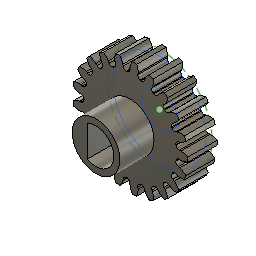
RS6-0845 Gear 21 Teeth HP9000 Laser Fusor v3 (Autodesk Fusion 360 design; units mm, degrees)
description: Spur Gear; Module: 1.024000; Num Teeth: 21; Pressure Angle: 14.500000; Backlash: 0.00 mm
Autodesk Fusion 360 part; units mm, degrees
(part 1 of 3)
sketch "Sketch1" plane through (0, 0, 0) normal (0, 0, 1) x (1, 0, 0) in component "Spur Gear (21 teeth)"
  circle A0 centre (0, 0) radius 9.4724
  circle A1 centre (0, 0) radius 3.625
  dimension "d8" = 7.25
  measures "d8" diameter of A1
extrude "Extrude1" add sketch "Sketch1" along normal blind 4 in component "Spur Gear (21 teeth)"
sketch "Sketch2" plane through (0, 0, 0) normal (0, 0, 1) x (1, 0, 0) in component "Spur Gear (21 teeth)"
  spline S0 degree 5 poles (10.3759, -0.8355) (10.3799, -0.8358) (10.3878, -0.8363) (10.3997, -0.8368) (10.4155, -0.837) (10.4354, -0.8366) (10.4552, -0.8356) (10.4751, -0.8343) (10.495, -0.8328) (10.5149, -0.8312) (10.5348, -0.8295) (10.5547, -0.8276) (10.5746, -0.8256) (10.5946, -0.8232) (10.6145, -0.8207) (10.6345, -0.8178) (10.6544, -0.8148) (10.6744, -0.8116) (10.6943, -0.8083) (10.7143, -0.8048) (10.7343, -0.8012) (10.7542, -0.7975) (10.7742, -0.7936) (10.7942, -0.7895) (10.8142, -0.7853) (10.8341, -0.781) (10.8541, -0.7765) (10.8741, -0.7719) (10.894, -0.7671) (10.914, -0.7622) (10.934, -0.7572) (10.9539, -0.752) (10.9739, -0.7468) (10.9939, -0.7414) (11.0138, -0.7359) (11.0338, -0.7302) (11.0537, -0.7245) (11.0737, -0.7186) (11.0936, -0.7126) (11.1136, -0.7065) (11.1335, -0.7003) (11.1534, -0.694) (11.1733, -0.6875) (11.1933, -0.681) (11.2132, -0.6743) (11.2331, -0.6675) (11.253, -0.6607) (11.2729, -0.6537) (11.2928, -0.6466) (11.3126, -0.6394) (11.3325, -0.6321) (11.3524, -0.6247) (11.3722, -0.6172) (11.3921, -0.6096) (11.4119, -0.6019) (11.4318, -0.5941) (11.4516, -0.5862) (11.4714, -0.5782) (11.4912, -0.5701) (11.511, -0.5619) (11.5308, -0.5536) (11.5506, -0.5452) (11.5704, -0.5367) (11.5901, -0.5281) (11.6099, -0.5194) (11.6296, -0.5106) (11.6494, -0.5018) (11.6691, -0.4928) (11.6888, -0.4838) (11.7085, -0.4746) (11.7282, -0.4654) (11.7439, -0.4579) (11.7557, -0.4523) (11.7636, -0.4485) (11.7675, -0.4466) knots 0 0 0 0 0 0 0.01428571 0.02857143 0.04285714 0.05714286 0.07142857 0.08571429 0.1 0.11428571 0.12857143 0.14285714 0.15714286 0.17142857 0.18571429 0.2 0.21428571 0.22857143 0.24285714 0.25714286 0.27142857 0.28571429 0.3 0.31428571 0.32857143 0.34285714 0.35714286 0.37142857 0.38571429 0.4 0.41428571 0.42857143 0.44285714 0.45714286 0.47142857 0.48571429 0.5 0.51428571 0.52857143 0.54285714 0.55714286 0.57142857 0.58571429 0.6 0.61428571 0.62857143 0.64285714 0.65714286 0.67142857 0.68571429 0.7 0.71428571 0.72857143 0.74285714 0.75714286 0.77142857 0.78571429 0.8 0.81428571 0.82857143 0.84285714 0.85714286 0.87142857 0.88571429 0.9 0.91428571 0.92857143 0.94285714 0.95714286 0.97142857 0.98571429 1 1 1 1 1 1
  spline S1 degree 5 poles (10.3759, 0.8355) (10.3799, 0.8358) (10.3878, 0.8363) (10.3997, 0.8368) (10.4155, 0.837) (10.4354, 0.8366) (10.4552, 0.8356) (10.4751, 0.8343) (10.495, 0.8328) (10.5149, 0.8312) (10.5348, 0.8295) (10.5547, 0.8276) (10.5746, 0.8256) (10.5946, 0.8232) (10.6145, 0.8207) (10.6345, 0.8178) (10.6544, 0.8148) (10.6744, 0.8116) (10.6943, 0.8083) (10.7143, 0.8048) (10.7343, 0.8012) (10.7542, 0.7975) (10.7742, 0.7936) (10.7942, 0.7895) (10.8142, 0.7853) (10.8341, 0.781) (10.8541, 0.7765) (10.8741, 0.7719) (10.894, 0.7671) (10.914, 0.7622) (10.934, 0.7572) (10.9539, 0.752) (10.9739, 0.7468) (10.9939, 0.7414) (11.0138, 0.7359) (11.0338, 0.7302) (11.0537, 0.7245) (11.0737, 0.7186) (11.0936, 0.7126) (11.1136, 0.7065) (11.1335, 0.7003) (11.1534, 0.694) (11.1733, 0.6875) (11.1933, 0.681) (11.2132, 0.6743) (11.2331, 0.6675) (11.253, 0.6607) (11.2729, 0.6537) (11.2928, 0.6466) (11.3126, 0.6394) (11.3325, 0.6321) (11.3524, 0.6247) (11.3722, 0.6172) (11.3921, 0.6096) (11.4119, 0.6019) (11.4318, 0.5941) (11.4516, 0.5862) (11.4714, 0.5782) (11.4912, 0.5701) (11.511, 0.5619) (11.5308, 0.5536) (11.5506, 0.5452) (11.5704, 0.5367) (11.5901, 0.5281) (11.6099, 0.5194) (11.6296, 0.5106) (11.6494, 0.5018) (11.6691, 0.4928) (11.6888, 0.4838) (11.7085, 0.4746) (11.7282, 0.4654) (11.7439, 0.4579) (11.7557, 0.4523) (11.7636, 0.4485) (11.7675, 0.4466) knots 0 0 0 0 0 0 0.01428571 0.02857143 0.04285714 0.05714286 0.07142857 0.08571429 0.1 0.11428571 0.12857143 0.14285714 0.15714286 0.17142857 0.18571429 0.2 0.21428571 0.22857143 0.24285714 0.25714286 0.27142857 0.28571429 0.3 0.31428571 0.32857143 0.34285714 0.35714286 0.37142857 0.38571429 0.4 0.41428571 0.42857143 0.44285714 0.45714286 0.47142857 0.48571429 0.5 0.51428571 0.52857143 0.54285714 0.55714286 0.57142857 0.58571429 0.6 0.61428571 0.62857143 0.64285714 0.65714286 0.67142857 0.68571429 0.7 0.71428571 0.72857143 0.74285714 0.75714286 0.77142857 0.78571429 0.8 0.81428571 0.82857143 0.84285714 0.85714286 0.87142857 0.88571429 0.9 0.91428571 0.92857143 0.94285714 0.95714286 0.97142857 0.98571429 1 1 1 1 1 1
  arc A0 (11.7675, -0.4466) -> (11.7675, 0.4466) centre (0, 0) ccw
  line L0 (9.4319, -0.7602) -> (10.3759, -0.8355)
  line L1 (9.4319, 0.7602) -> (10.3759, 0.8355)
  line L2 (9.4319, -0.7602) -> (9.4319, 0.7602)
  point P0 (10.4739, -0.8344)
  point P1 (10.5725, -0.8257)
  point P2 (10.6715, -0.8121)
  point P3 (10.7707, -0.7943)
  point P4 (10.8701, -0.7727)
  point P5 (10.9697, -0.7479)
  point P6 (11.0694, -0.7198)
  point P7 (11.1691, -0.6889)
  point P8 (11.269, -0.655)
  point P9 (11.3688, -0.6185)
  point P10 (11.4686, -0.5793)
  point P11 (11.5683, -0.5376)
  point P12 (11.668, -0.4933)
  point P13 (10.4739, 0.8344)
  point P14 (10.5725, 0.8257)
  point P15 (10.6715, 0.8121)
  point P16 (10.7707, 0.7943)
  point P17 (10.8701, 0.7727)
  point P18 (10.9697, 0.7479)
  point P19 (11.0694, 0.7198)
  point P20 (11.1691, 0.6889)
  point P21 (11.269, 0.655)
  point P22 (11.3688, 0.6185)
  point P23 (11.4686, 0.5793)
  point P24 (11.5683, 0.5376)
  point P25 (11.668, 0.4933)
extrude "Extrude2" add sketch "Sketch2" along normal blind 4 in component "Spur Gear (21 teeth)"
fillet "Fillet1" radius 0.62 2 edges at (9.4418, -0.761, 2) (9.4418, 0.761, 2) in component "Spur Gear (21 teeth)"
pattern_circular "C-Pattern1" count 21 over 360 about axis through (0, 0, 0) along (0, 0, 1) of "Extrude2", "Fillet1" in component "Spur Gear (21 teeth)"
sketch "Sketch3" plane through (0, 0, 0) normal (0, 0, 1) x (1, 0, 0) in component "Spur Gear (21 teeth)"
  circle A0 centre (0, 0) radius 10.752 construction
sketch "Sketch1 (2)" plane through (0, 0, 0) normal (0, 0, 1) x (1, 0, 0)
  circle A0 centre (0, 0) radius 3.625
  line L0 (-1.775, 0) -> (-1.775, 3.1607)
  line L1 (-1.775, 0) -> (-1.775, -3.1607)
  point P0 (-3.625, 0)
  dimension "d9" = 1.85
  constraint coincident A0.centre origin
  constraint vertical L0
  constraint coincident A0 L0.end
  constraint vertical L1
  constraint coincident A0 L1.end
  measures "d9" distance of P0 L0.start
extrude "Extrude3" add 1 faces at (2.7368, -6.9731, 4) along direction (0, 0, 1) blind 3 in component "Spur Gear (21 teeth)"
sketch "Sketch2 (2)" plane through (0, 0, 7) normal (0, 0, 1) x (1, 0, 0)
  arc A0 (9.3554, -1.4844) -> (9.3773, -1.3391) centre (0, 0) ccw
  arc A1 (10.0403, -0.8087) -> (9.3773, -1.3391) centre (9.991, -1.4268) ccw
  line L0 (10.0403, -0.8087) -> (10.3759, -0.8355)
  spline S0 degree 5 poles (10.3759, -0.8355) (10.3799, -0.8358) (10.3878, -0.8363) (10.3997, -0.8368) (10.4155, -0.837) (10.4354, -0.8366) (10.4552, -0.8356) (10.4751, -0.8343) (10.495, -0.8328) (10.5149, -0.8312) (10.5348, -0.8295) (10.5547, -0.8276) (10.5746, -0.8256) (10.5946, -0.8232) (10.6145, -0.8207) (10.6345, -0.8178) (10.6544, -0.8148) (10.6744, -0.8116) (10.6943, -0.8083) (10.7143, -0.8048) (10.7343, -0.8012) (10.7542, -0.7975) (10.7742, -0.7936) (10.7942, -0.7895) (10.8142, -0.7853) (10.8341, -0.781) (10.8541, -0.7765) (10.8741, -0.7719) (10.894, -0.7671) (10.914, -0.7622) (10.934, -0.7572) (10.9539, -0.752) (10.9739, -0.7468) (10.9939, -0.7414) (11.0138, -0.7359) (11.0338, -0.7302) (11.0537, -0.7245) (11.0737, -0.7186) (11.0936, -0.7126) (11.1136, -0.7065) (11.1335, -0.7003) (11.1534, -0.694) (11.1733, -0.6875) (11.1933, -0.681) (11.2132, -0.6743) (11.2331, -0.6675) (11.253, -0.6607) (11.2729, -0.6537) (11.2928, -0.6466) (11.3126, -0.6394) (11.3325, -0.6321) (11.3524, -0.6247) (11.3722, -0.6172) (11.3921, -0.6096) (11.4119, -0.6019) (11.4318, -0.5941) (11.4516, -0.5862) (11.4714, -0.5782) (11.4912, -0.5701) (11.511, -0.5619) (11.5308, -0.5536) (11.5506, -0.5452) (11.5704, -0.5367) (11.5901, -0.5281) (11.6099, -0.5194) (11.6296, -0.5106) (11.6494, -0.5018) (11.6691, -0.4928) (11.6888, -0.4838) (11.7085, -0.4746) (11.7282, -0.4654) (11.7439, -0.4579) (11.7557, -0.4523) (11.7636, -0.4485) (11.7675, -0.4466) knots 0 0 0 0 0 0 0.01428571 0.02857143 0.04285714 0.05714286 0.07142857 0.08571429 0.1 0.11428571 0.12857143 0.14285714 0.15714286 0.17142857 0.18571429 0.2 0.21428571 0.22857143 0.24285714 0.25714286 0.27142857 0.28571429 0.3 0.31428571 0.32857143 0.34285714 0.35714286 0.37142857 0.38571429 0.4 0.41428571 0.42857143 0.44285714 0.45714286 0.47142857 0.48571429 0.5 0.51428571 0.52857143 0.54285714 0.55714286 0.57142857 0.58571429 0.6 0.61428571 0.62857143 0.64285714 0.65714286 0.67142857 0.68571429 0.7 0.71428571 0.72857143 0.74285714 0.75714286 0.77142857 0.78571429 0.8 0.81428571 0.82857143 0.84285714 0.85714286 0.87142857 0.88571429 0.9 0.91428571 0.92857143 0.94285714 0.95714286 0.97142857 0.98571429 1 1 1 1 1 1
  arc A2 (11.7675, -0.4466) -> (11.7675, 0.4466) centre (0, 0) ccw
  spline S1 degree 5 poles (11.7675, 0.4466) (11.7636, 0.4485) (11.7557, 0.4523) (11.7439, 0.4579) (11.7282, 0.4654) (11.7085, 0.4746) (11.6888, 0.4838) (11.6691, 0.4928) (11.6494, 0.5018) (11.6296, 0.5106) (11.6099, 0.5194) (11.5901, 0.5281) (11.5704, 0.5367) (11.5506, 0.5452) (11.5308, 0.5536) (11.511, 0.5619) (11.4912, 0.5701) (11.4714, 0.5782) (11.4516, 0.5862) (11.4318, 0.5941) (11.4119, 0.6019) (11.3921, 0.6096) (11.3722, 0.6172) (11.3524, 0.6247) (11.3325, 0.6321) (11.3126, 0.6394) (11.2928, 0.6466) (11.2729, 0.6537) (11.253, 0.6607) (11.2331, 0.6675) (11.2132, 0.6743) (11.1933, 0.681) (11.1733, 0.6875) (11.1534, 0.694) (11.1335, 0.7003) (11.1136, 0.7065) (11.0936, 0.7126) (11.0737, 0.7186) (11.0537, 0.7245) (11.0338, 0.7302) (11.0138, 0.7359) (10.9939, 0.7414) (10.9739, 0.7468) (10.9539, 0.752) (10.934, 0.7572) (10.914, 0.7622) (10.894, 0.7671) (10.8741, 0.7719) (10.8541, 0.7765) (10.8341, 0.781) (10.8142, 0.7853) (10.7942, 0.7895) (10.7742, 0.7936) (10.7542, 0.7975) (10.7343, 0.8012) (10.7143, 0.8048) (10.6943, 0.8083) (10.6744, 0.8116) (10.6544, 0.8148) (10.6345, 0.8178) (10.6145, 0.8207) (10.5946, 0.8232) (10.5746, 0.8256) (10.5547, 0.8276) (10.5348, 0.8295) (10.5149, 0.8312) (10.495, 0.8328) (10.4751, 0.8343) (10.4552, 0.8356) (10.4354, 0.8366) (10.4155, 0.837) (10.3997, 0.8368) (10.3878, 0.8363) (10.3799, 0.8358) (10.3759, 0.8355) knots -1 -1 -1 -1 -1 -1 -0.98571429 -0.97142857 -0.95714286 -0.94285714 -0.92857143 -0.91428571 -0.9 -0.88571429 -0.87142857 -0.85714286 -0.84285714 -0.82857143 -0.81428571 -0.8 -0.78571429 -0.77142857 -0.75714286 -0.74285714 -0.72857143 -0.71428571 -0.7 -0.68571429 -0.67142857 -0.65714286 -0.64285714 -0.62857143 -0.61428571 -0.6 -0.58571429 -0.57142857 -0.55714286 -0.54285714 -0.52857143 -0.51428571 -0.5 -0.48571429 -0.47142857 -0.45714286 -0.44285714 -0.42857143 -0.41428571 -0.4 -0.38571429 -0.37142857 -0.35714286 -0.34285714 -0.32857143 -0.31428571 -0.3 -0.28571429 -0.27142857 -0.25714286 -0.24285714 -0.22857143 -0.21428571 -0.2 -0.18571429 -0.17142857 -0.15714286 -0.14285714 -0.12857143 -0.11428571 -0.1 -0.08571429 -0.07142857 -0.05714286 -0.04285714 -0.02857143 -0.01428571 0 0 0 0 0 0
  line L1 (10.3759, 0.8355) -> (10.0403, 0.8087)
  arc A3 (9.3773, 1.3391) -> (10.0403, 0.8087) centre (9.991, 1.4268) ccw
  arc A4 (9.3773, 1.3391) -> (9.3554, 1.4844) centre (0, 0) ccw
  arc A5 (9.8326, 2.1866) -> (9.3554, 1.4844) centre (9.9677, 1.5815) ccw
  line L2 (9.8326, 2.1866) -> (10.1612, 2.26)
  spline S2 degree 5 poles (10.1612, 2.26) (10.1651, 2.2609) (10.1728, 2.2627) (10.1843, 2.2657) (10.1995, 2.2702) (10.2183, 2.2765) (10.237, 2.2832) (10.2556, 2.2903) (10.2742, 2.2976) (10.2928, 2.305) (10.3113, 2.3125) (10.3298, 2.3202) (10.3482, 2.328) (10.3665, 2.3361) (10.3848, 2.3445) (10.4031, 2.3531) (10.4213, 2.3618) (10.4394, 2.3707) (10.4575, 2.3798) (10.4755, 2.389) (10.4936, 2.3983) (10.5115, 2.4078) (10.5295, 2.4174) (10.5474, 2.4272) (10.5652, 2.4371) (10.583, 2.4471) (10.6008, 2.4573) (10.6185, 2.4676) (10.6362, 2.4781) (10.6538, 2.4886) (10.6714, 2.4993) (10.689, 2.5101) (10.7065, 2.521) (10.724, 2.532) (10.7414, 2.5432) (10.7588, 2.5545) (10.7762, 2.5659) (10.7935, 2.5773) (10.8108, 2.5889) (10.8281, 2.6007) (10.8453, 2.6125) (10.8624, 2.6244) (10.8796, 2.6364) (10.8967, 2.6486) (10.9138, 2.6608) (10.9308, 2.6731) (10.9478, 2.6856) (10.9647, 2.6981) (10.9816, 2.7107) (10.9985, 2.7235) (11.0154, 2.7363) (11.0322, 2.7492) (11.0489, 2.7623) (11.0657, 2.7754) (11.0823, 2.7886) (11.099, 2.8019) (11.1156, 2.8153) (11.1322, 2.8288) (11.1487, 2.8424) (11.1652, 2.856) (11.1817, 2.8698) (11.1981, 2.8837) (11.2145, 2.8976) (11.2309, 2.9116) (11.2472, 2.9257) (11.2635, 2.9399) (11.2797, 2.9542) (11.2959, 2.9686) (11.3121, 2.9831) (11.3282, 2.9976) (11.3443, 3.0122) (11.3572, 3.024) (11.3668, 3.0329) (11.3732, 3.0388) (11.3764, 3.0418) knots 0 0 0 0 0 0 0.01428571 0.02857143 0.04285714 0.05714286 0.07142857 0.08571429 0.1 0.11428571 0.12857143 0.14285714 0.15714286 0.17142857 0.18571429 0.2 0.21428571 0.22857143 0.24285714 0.25714286 0.27142857 0.28571429 0.3 0.31428571 0.32857143 0.34285714 0.35714286 0.37142857 0.38571429 0.4 0.41428571 0.42857143 0.44285714 0.45714286 0.47142857 0.48571429 0.5 0.51428571 0.52857143 0.54285714 0.55714286 0.57142857 0.58571429 0.6 0.61428571 0.62857143 0.64285714 0.65714286 0.67142857 0.68571429 0.7 0.71428571 0.72857143 0.74285714 0.75714286 0.77142857 0.78571429 0.8 0.81428571 0.82857143 0.84285714 0.85714286 0.87142857 0.88571429 0.9 0.91428571 0.92857143 0.94285714 0.95714286 0.97142857 0.98571429 1 1 1 1 1 1
  arc A6 (11.3764, 3.0418) -> (11.1131, 3.8953) centre (0, 0) ccw
  spline S3 degree 5 poles (11.1131, 3.8953) (11.1088, 3.896) (11.1001, 3.8973) (11.0872, 3.8992) (11.07, 3.9017) (11.0484, 3.9047) (11.0269, 3.9076) (11.0054, 3.9105) (10.9839, 3.9132) (10.9625, 3.9159) (10.941, 3.9184) (10.9196, 3.9209) (10.8982, 3.9233) (10.8768, 3.9256) (10.8554, 3.9277) (10.834, 3.9298) (10.8127, 3.9318) (10.7914, 3.9337) (10.7701, 3.9355) (10.7488, 3.9373) (10.7275, 3.9389) (10.7063, 3.9404) (10.6851, 3.9418) (10.6639, 3.9431) (10.6427, 3.9443) (10.6216, 3.9454) (10.6005, 3.9465) (10.5794, 3.9474) (10.5583, 3.9482) (10.5373, 3.9489) (10.5162, 3.9495) (10.4953, 3.95) (10.4743, 3.9504) (10.4534, 3.9507) (10.4324, 3.9508) (10.4116, 3.9509) (10.3907, 3.9509) (10.3699, 3.9507) (10.3491, 3.9504) (10.3283, 3.9501) (10.3076, 3.9496) (10.2869, 3.9489) (10.2662, 3.9482) (10.2456, 3.9474) (10.225, 3.9464) (10.2045, 3.9453) (10.1839, 3.9441) (10.1635, 3.9427) (10.143, 3.9413) (10.1226, 3.9397) (10.1022, 3.938) (10.0819, 3.9361) (10.0616, 3.9341) (10.0414, 3.9319) (10.0212, 3.9296) (10.0011, 3.9272) (9.981, 3.9246) (9.9609, 3.9219) (9.9409, 3.9191) (9.921, 3.9161) (9.9011, 3.9129) (9.8812, 3.9095) (9.8615, 3.9058) (9.8418, 3.9019) (9.8223, 3.8979) (9.8027, 3.8936) (9.7832, 3.8893) (9.7638, 3.8848) (9.7444, 3.8802) (9.7252, 3.8753) (9.7061, 3.8699) (9.691, 3.865) (9.6798, 3.861) (9.6724, 3.8582) (9.6687, 3.8567) knots -1 -1 -1 -1 -1 -1 -0.98571429 -0.97142857 -0.95714286 -0.94285714 -0.92857143 -0.91428571 -0.9 -0.88571429 -0.87142857 -0.85714286 -0.84285714 -0.82857143 -0.81428571 -0.8 -0.78571429 -0.77142857 -0.75714286 -0.74285714 -0.72857143 -0.71428571 -0.7 -0.68571429 -0.67142857 -0.65714286 -0.64285714 -0.62857143 -0.61428571 -0.6 -0.58571429 -0.57142857 -0.55714286 -0.54285714 -0.52857143 -0.51428571 -0.5 -0.48571429 -0.47142857 -0.45714286 -0.44285714 -0.42857143 -0.41428571 -0.4 -0.38571429 -0.37142857 -0.35714286 -0.34285714 -0.32857143 -0.31428571 -0.3 -0.28571429 -0.27142857 -0.25714286 -0.24285714 -0.22857143 -0.21428571 -0.2 -0.18571429 -0.17142857 -0.15714286 -0.14285714 -0.12857143 -0.11428571 -0.1 -0.08571429 -0.07142857 -0.05714286 -0.04285714 -0.02857143 -0.01428571 0 0 0 0 0 0
  line L3 (9.6687, 3.8567) -> (9.3558, 3.7322)
  arc A7 (8.566, 4.0436) -> (9.3558, 3.7322) centre (9.1266, 4.3083) ccw
  arc A8 (8.566, 4.0436) -> (8.5022, 4.176) centre (0, 0) ccw
  arc A9 (8.7512, 4.9877) -> (8.5022, 4.176) centre (9.0587, 4.4493) ccw
  line L4 (8.7512, 4.9877) -> (9.0436, 5.1547)
  spline S4 degree 5 poles (9.0436, 5.1547) (9.0471, 5.1567) (9.0539, 5.1607) (9.064, 5.1669) (9.0772, 5.1757) (9.0934, 5.1872) (9.1092, 5.1992) (9.1249, 5.2115) (9.1405, 5.2239) (9.1561, 5.2364) (9.1715, 5.2491) (9.1869, 5.2619) (9.2022, 5.2748) (9.2174, 5.288) (9.2324, 5.3013) (9.2473, 5.3149) (9.2621, 5.3286) (9.2768, 5.3425) (9.2914, 5.3565) (9.306, 5.3706) (9.3204, 5.3848) (9.3348, 5.3992) (9.3491, 5.4136) (9.3633, 5.4282) (9.3775, 5.443) (9.3915, 5.4578) (9.4055, 5.4728) (9.4194, 5.4878) (9.4332, 5.503) (9.4469, 5.5183) (9.4606, 5.5337) (9.4742, 5.5492) (9.4877, 5.5648) (9.5012, 5.5805) (9.5146, 5.5963) (9.5279, 5.6122) (9.5411, 5.6282) (9.5543, 5.6443) (9.5674, 5.6605) (9.5804, 5.6767) (9.5934, 5.6931) (9.6063, 5.7096) (9.6191, 5.7261) (9.6319, 5.7427) (9.6446, 5.7595) (9.6572, 5.7763) (9.6698, 5.7932) (9.6823, 5.8101) (9.6948, 5.8272) (9.7071, 5.8444) (9.7194, 5.8616) (9.7317, 5.8789) (9.7439, 5.8963) (9.756, 5.9137) (9.768, 5.9313) (9.78, 5.9489) (9.792, 5.9666) (9.8038, 5.9844) (9.8156, 6.0022) (9.8274, 6.0202) (9.8391, 6.0382) (9.8507, 6.0563) (9.8622, 6.0744) (9.8737, 6.0926) (9.8851, 6.1109) (9.8965, 6.1293) (9.9078, 6.1477) (9.9191, 6.1662) (9.9303, 6.1848) (9.9414, 6.2035) (9.9524, 6.2222) (9.9613, 6.2372) (9.9678, 6.2485) (9.9722, 6.2561) (9.9744, 6.2599) knots 0 0 0 0 0 0 0.01428571 0.02857143 0.04285714 0.05714286 0.07142857 0.08571429 0.1 0.11428571 0.12857143 0.14285714 0.15714286 0.17142857 0.18571429 0.2 0.21428571 0.22857143 0.24285714 0.25714286 0.27142857 0.28571429 0.3 0.31428571 0.32857143 0.34285714 0.35714286 0.37142857 0.38571429 0.4 0.41428571 0.42857143 0.44285714 0.45714286 0.47142857 0.48571429 0.5 0.51428571 0.52857143 0.54285714 0.55714286 0.57142857 0.58571429 0.6 0.61428571 0.62857143 0.64285714 0.65714286 0.67142857 0.68571429 0.7 0.71428571 0.72857143 0.74285714 0.75714286 0.77142857 0.78571429 0.8 0.81428571 0.82857143 0.84285714 0.85714286 0.87142857 0.88571429 0.9 0.91428571 0.92857143 0.94285714 0.95714286 0.97142857 0.98571429 1 1 1 1 1 1
  arc A10 (9.9744, 6.2599) -> (9.4712, 6.9979) centre (0, 0) ccw
  spline S5 degree 5 poles (9.4712, 6.9979) (9.4669, 6.9973) (9.4583, 6.9959) (9.4453, 6.994) (9.4281, 6.9912) (9.4067, 6.9878) (9.3852, 6.9842) (9.3638, 6.9806) (9.3425, 6.9769) (9.3212, 6.9731) (9.3, 6.9693) (9.2787, 6.9653) (9.2576, 6.9613) (9.2365, 6.9571) (9.2154, 6.9529) (9.1944, 6.9486) (9.1734, 6.9442) (9.1524, 6.9398) (9.1316, 6.9352) (9.1107, 6.9306) (9.0899, 6.9259) (9.0692, 6.9211) (9.0485, 6.9162) (9.0279, 6.9112) (9.0073, 6.9061) (8.9868, 6.9009) (8.9663, 6.8957) (8.9459, 6.8903) (8.9255, 6.8849) (8.9052, 6.8794) (8.8849, 6.8737) (8.8647, 6.868) (8.8446, 6.8622) (8.8245, 6.8563) (8.8044, 6.8503) (8.7845, 6.8442) (8.7645, 6.838) (8.7447, 6.8318) (8.7249, 6.8254) (8.7052, 6.8189) (8.6855, 6.8123) (8.6659, 6.8056) (8.6464, 6.7988) (8.6269, 6.7919) (8.6075, 6.7849) (8.5882, 6.7778) (8.569, 6.7706) (8.5498, 6.7633) (8.5307, 6.7559) (8.5116, 6.7484) (8.4927, 6.7407) (8.4738, 6.7329) (8.455, 6.725) (8.4363, 6.717) (8.4177, 6.7089) (8.3992, 6.7006) (8.3807, 6.6922) (8.3624, 6.6837) (8.3441, 6.6751) (8.3259, 6.6663) (8.3078, 6.6574) (8.2899, 6.6483) (8.2721, 6.639) (8.2545, 6.6295) (8.237, 6.6198) (8.2195, 6.6101) (8.2022, 6.6002) (8.1849, 6.5902) (8.1678, 6.5801) (8.1508, 6.5697) (8.1342, 6.5589) (8.1212, 6.5498) (8.1117, 6.5426) (8.1055, 6.5377) (8.1024, 6.5353) knots -1 -1 -1 -1 -1 -1 -0.98571429 -0.97142857 -0.95714286 -0.94285714 -0.92857143 -0.91428571 -0.9 -0.88571429 -0.87142857 -0.85714286 -0.84285714 -0.82857143 -0.81428571 -0.8 -0.78571429 -0.77142857 -0.75714286 -0.74285714 -0.72857143 -0.71428571 -0.7 -0.68571429 -0.67142857 -0.65714286 -0.64285714 -0.62857143 -0.61428571 -0.6 -0.58571429 -0.57142857 -0.55714286 -0.54285714 -0.52857143 -0.51428571 -0.5 -0.48571429 -0.47142857 -0.45714286 -0.44285714 -0.42857143 -0.41428571 -0.4 -0.38571429 -0.37142857 -0.35714286 -0.34285714 -0.32857143 -0.31428571 -0.3 -0.28571429 -0.27142857 -0.25714286 -0.24285714 -0.22857143 -0.21428571 -0.2 -0.18571429 -0.17142857 -0.15714286 -0.14285714 -0.12857143 -0.11428571 -0.1 -0.08571429 -0.07142857 -0.05714286 -0.04285714 -0.02857143 -0.01428571 0 0 0 0 0 0
  line L5 (8.1024, 6.5353) -> (7.8401, 6.3241)
  arc A11 (6.9935, 6.3888) -> (7.8401, 6.3241) centre (7.4513, 6.807) ccw
  arc A12 (6.9935, 6.3888) -> (6.8936, 6.4965) centre (0, 0) ccw
  arc A13 (6.8923, 7.3456) -> (6.8936, 6.4965) centre (7.3448, 6.9217) ccw
  line L6 (6.8923, 7.3456) -> (7.1225, 7.5913)
  spline S6 degree 5 poles (7.1225, 7.5913) (7.1252, 7.5942) (7.1305, 7.6001) (7.1384, 7.609) (7.1484, 7.6213) (7.1604, 7.6371) (7.172, 7.6532) (7.1834, 7.6696) (7.1947, 7.686) (7.2058, 7.7026) (7.2169, 7.7192) (7.2278, 7.736) (7.2386, 7.7529) (7.2492, 7.7699) (7.2597, 7.7871) (7.2699, 7.8044) (7.28, 7.8219) (7.2899, 7.8395) (7.2998, 7.8572) (7.3095, 7.875) (7.3191, 7.8928) (7.3287, 7.9108) (7.3381, 7.9288) (7.3474, 7.947) (7.3565, 7.9652) (7.3656, 7.9835) (7.3745, 8.0019) (7.3833, 8.0204) (7.3921, 8.039) (7.4007, 8.0577) (7.4092, 8.0764) (7.4176, 8.0952) (7.426, 8.1141) (7.4342, 8.1331) (7.4423, 8.1521) (7.4504, 8.1713) (7.4583, 8.1904) (7.4661, 8.2097) (7.4739, 8.229) (7.4816, 8.2484) (7.4891, 8.2679) (7.4966, 8.2874) (7.504, 8.307) (7.5113, 8.3267) (7.5185, 8.3464) (7.5256, 8.3662) (7.5326, 8.386) (7.5396, 8.4059) (7.5464, 8.4259) (7.5532, 8.4459) (7.5599, 8.466) (7.5665, 8.4862) (7.573, 8.5064) (7.5794, 8.5266) (7.5858, 8.547) (7.5921, 8.5673) (7.5982, 8.5878) (7.6043, 8.6082) (7.6104, 8.6288) (7.6163, 8.6494) (7.6221, 8.67) (7.6279, 8.6907) (7.6336, 8.7115) (7.6392, 8.7323) (7.6448, 8.7531) (7.6502, 8.774) (7.6556, 8.795) (7.6609, 8.816) (7.6661, 8.837) (7.6712, 8.8582) (7.6763, 8.8793) (7.6802, 8.8963) (7.6832, 8.909) (7.6851, 8.9175) (7.6861, 8.9218) knots 0 0 0 0 0 0 0.01428571 0.02857143 0.04285714 0.05714286 0.07142857 0.08571429 0.1 0.11428571 0.12857143 0.14285714 0.15714286 0.17142857 0.18571429 0.2 0.21428571 0.22857143 0.24285714 0.25714286 0.27142857 0.28571429 0.3 0.31428571 0.32857143 0.34285714 0.35714286 0.37142857 0.38571429 0.4 0.41428571 0.42857143 0.44285714 0.45714286 0.47142857 0.48571429 0.5 0.51428571 0.52857143 0.54285714 0.55714286 0.57142857 0.58571429 0.6 0.61428571 0.62857143 0.64285714 0.65714286 0.67142857 0.68571429 0.7 0.71428571 0.72857143 0.74285714 0.75714286 0.77142857 0.78571429 0.8 0.81428571 0.82857143 0.84285714 0.85714286 0.87142857 0.88571429 0.9 0.91428571 0.92857143 0.94285714 0.95714286 0.97142857 0.98571429 1 1 1 1 1 1
  arc A14 (7.6861, 8.9218) -> (6.9877, 9.4787) centre (0, 0) ccw
  spline S7 degree 5 poles (6.9877, 9.4787) (6.9838, 9.4768) (6.976, 9.473) (6.9642, 9.4673) (6.9485, 9.4596) (6.9291, 9.45) (6.9096, 9.4403) (6.8903, 9.4305) (6.871, 9.4207) (6.8517, 9.4108) (6.8326, 9.4008) (6.8135, 9.3908) (6.7944, 9.3807) (6.7755, 9.3705) (6.7566, 9.3603) (6.7377, 9.35) (6.719, 9.3396) (6.7003, 9.3292) (6.6817, 9.3187) (6.6631, 9.3081) (6.6447, 9.2975) (6.6263, 9.2868) (6.6079, 9.276) (6.5897, 9.2651) (6.5715, 9.2542) (6.5534, 9.2432) (6.5354, 9.2322) (6.5175, 9.221) (6.4996, 9.2098) (6.4818, 9.1986) (6.4641, 9.1872) (6.4465, 9.1758) (6.4289, 9.1643) (6.4115, 9.1528) (6.3941, 9.1411) (6.3768, 9.1294) (6.3596, 9.1176) (6.3425, 9.1058) (6.3255, 9.0939) (6.3085, 9.0818) (6.2917, 9.0698) (6.2749, 9.0576) (6.2583, 9.0453) (6.2417, 9.033) (6.2252, 9.0206) (6.2089, 9.0081) (6.1926, 8.9956) (6.1764, 8.9829) (6.1603, 8.9702) (6.1444, 8.9574) (6.1285, 8.9445) (6.1128, 8.9315) (6.0972, 8.9184) (6.0817, 8.9052) (6.0663, 8.892) (6.051, 8.8786) (6.0359, 8.8652) (6.0208, 8.8516) (6.0059, 8.838) (5.9911, 8.8243) (5.9764, 8.8104) (5.962, 8.7965) (5.9477, 8.7823) (5.9337, 8.768) (5.9198, 8.7536) (5.906, 8.7391) (5.8924, 8.7246) (5.8788, 8.7099) (5.8654, 8.6952) (5.8523, 8.6803) (5.8395, 8.6651) (5.8298, 8.6526) (5.8228, 8.6429) (5.8183, 8.6364) (5.8161, 8.6331) knots -1 -1 -1 -1 -1 -1 -0.98571429 -0.97142857 -0.95714286 -0.94285714 -0.92857143 -0.91428571 -0.9 -0.88571429 -0.87142857 -0.85714286 -0.84285714 -0.82857143 -0.81428571 -0.8 -0.78571429 -0.77142857 -0.75714286 -0.74285714 -0.72857143 -0.71428571 -0.7 -0.68571429 -0.67142857 -0.65714286 -0.64285714 -0.62857143 -0.61428571 -0.6 -0.58571429 -0.57142857 -0.55714286 -0.54285714 -0.52857143 -0.51428571 -0.5 -0.48571429 -0.47142857 -0.45714286 -0.44285714 -0.42857143 -0.41428571 -0.4 -0.38571429 -0.37142857 -0.35714286 -0.34285714 -0.32857143 -0.31428571 -0.3 -0.28571429 -0.27142857 -0.25714286 -0.24285714 -0.22857143 -0.21428571 -0.2 -0.18571429 -0.17142857 -0.15714286 -0.14285714 -0.12857143 -0.11428571 -0.1 -0.08571429 -0.07142857 -0.05714286 -0.04285714 -0.02857143 -0.01428571 0 0 0 0 0 0
  line L7 (5.8161, 8.6331) -> (5.6277, 8.354)
  arc A15 (4.7997, 8.1664) -> (5.6277, 8.354) centre (5.1138, 8.7009) ccw
  arc A16 (4.7997, 8.1664) -> (4.6724, 8.2398) centre (0, 0) ccw
  arc A17 (4.4209, 9.0508) -> (4.6724, 8.2398) centre (4.9783, 8.7791) ccw
  line L8 (4.4209, 9.0508) -> (4.5685, 9.3535)
  spline S8 degree 5 poles (4.5685, 9.3535) (4.5702, 9.357) (4.5736, 9.3642) (4.5784, 9.375) (4.5844, 9.3897) (4.5912, 9.4084) (4.5976, 9.4272) (4.6036, 9.4462) (4.6095, 9.4652) (4.6153, 9.4843) (4.621, 9.5035) (4.6265, 9.5227) (4.6318, 9.542) (4.637, 9.5615) (4.6418, 9.581) (4.6465, 9.6006) (4.651, 9.6202) (4.6553, 9.64) (4.6595, 9.6598) (4.6636, 9.6796) (4.6675, 9.6995) (4.6713, 9.7195) (4.675, 9.7395) (4.6785, 9.7596) (4.6819, 9.7797) (4.6851, 9.7999) (4.6883, 9.8201) (4.6912, 9.8404) (4.6941, 9.8607) (4.6968, 9.8811) (4.6995, 9.9015) (4.702, 9.922) (4.7044, 9.9425) (4.7066, 9.963) (4.7088, 9.9836) (4.7108, 10.0043) (4.7128, 10.0249) (4.7146, 10.0457) (4.7163, 10.0664) (4.7179, 10.0872) (4.7194, 10.108) (4.7208, 10.1289) (4.7221, 10.1498) (4.7233, 10.1707) (4.7243, 10.1917) (4.7253, 10.2127) (4.7262, 10.2337) (4.7269, 10.2548) (4.7276, 10.2759) (4.7282, 10.297) (4.7286, 10.3182) (4.729, 10.3394) (4.7293, 10.3606) (4.7294, 10.3819) (4.7295, 10.4032) (4.7295, 10.4245) (4.7294, 10.4459) (4.7292, 10.4672) (4.7289, 10.4886) (4.7285, 10.5101) (4.728, 10.5315) (4.7274, 10.553) (4.7267, 10.5745) (4.7259, 10.596) (4.7251, 10.6176) (4.7241, 10.6392) (4.7231, 10.6608) (4.722, 10.6824) (4.7207, 10.7041) (4.7194, 10.7257) (4.718, 10.7474) (4.7168, 10.7648) (4.7159, 10.7779) (4.7152, 10.7866) (4.7149, 10.7909) knots 0 0 0 0 0 0 0.01428571 0.02857143 0.04285714 0.05714286 0.07142857 0.08571429 0.1 0.11428571 0.12857143 0.14285714 0.15714286 0.17142857 0.18571429 0.2 0.21428571 0.22857143 0.24285714 0.25714286 0.27142857 0.28571429 0.3 0.31428571 0.32857143 0.34285714 0.35714286 0.37142857 0.38571429 0.4 0.41428571 0.42857143 0.44285714 0.45714286 0.47142857 0.48571429 0.5 0.51428571 0.52857143 0.54285714 0.55714286 0.57142857 0.58571429 0.6 0.61428571 0.62857143 0.64285714 0.65714286 0.67142857 0.68571429 0.7 0.71428571 0.72857143 0.74285714 0.75714286 0.77142857 0.78571429 0.8 0.81428571 0.82857143 0.84285714 0.85714286 0.87142857 0.88571429 0.9 0.91428571 0.92857143 0.94285714 0.95714286 0.97142857 0.98571429 1 1 1 1 1 1
  arc A18 (4.7149, 10.7909) -> (3.8834, 11.1173) centre (0, 0) ccw
  spline S9 degree 5 poles (3.8834, 11.1173) (3.8802, 11.1143) (3.8738, 11.1083) (3.8643, 11.0994) (3.8516, 11.0875) (3.8358, 11.0725) (3.8201, 11.0575) (3.8044, 11.0425) (3.7889, 11.0274) (3.7734, 11.0123) (3.7581, 10.9971) (3.7428, 10.9819) (3.7276, 10.9666) (3.7124, 10.9513) (3.6974, 10.936) (3.6824, 10.9206) (3.6676, 10.9052) (3.6528, 10.8897) (3.6381, 10.8742) (3.6235, 10.8586) (3.609, 10.843) (3.5946, 10.8273) (3.5802, 10.8116) (3.566, 10.7959) (3.5518, 10.7801) (3.5378, 10.7642) (3.5238, 10.7484) (3.51, 10.7324) (3.4962, 10.7165) (3.4825, 10.7005) (3.4689, 10.6844) (3.4555, 10.6683) (3.4421, 10.6521) (3.4288, 10.636) (3.4156, 10.6197) (3.4026, 10.6034) (3.3896, 10.5871) (3.3767, 10.5707) (3.364, 10.5543) (3.3513, 10.5378) (3.3388, 10.5213) (3.3264, 10.5048) (3.3141, 10.4881) (3.3019, 10.4715) (3.2898, 10.4548) (3.2778, 10.438) (3.266, 10.4212) (3.2542, 10.4044) (3.2426, 10.3875) (3.2312, 10.3705) (3.2198, 10.3535) (3.2086, 10.3365) (3.1975, 10.3194) (3.1866, 10.3022) (3.1758, 10.285) (3.1652, 10.2677) (3.1546, 10.2504) (3.1443, 10.233) (3.134, 10.2156) (3.1239, 10.1981) (3.114, 10.1806) (3.1043, 10.163) (3.0949, 10.1453) (3.0856, 10.1275) (3.0766, 10.1096) (3.0677, 10.0917) (3.059, 10.0738) (3.0503, 10.0558) (3.0419, 10.0378) (3.0337, 10.0196) (3.026, 10.0013) (3.0204, 9.9865) (3.0166, 9.9753) (3.0142, 9.9677) (3.0131, 9.9639) knots -1 -1 -1 -1 -1 -1 -0.98571429 -0.97142857 -0.95714286 -0.94285714 -0.92857143 -0.91428571 -0.9 -0.88571429 -0.87142857 -0.85714286 -0.84285714 -0.82857143 -0.81428571 -0.8 -0.78571429 -0.77142857 -0.75714286 -0.74285714 -0.72857143 -0.71428571 -0.7 -0.68571429 -0.67142857 -0.65714286 -0.64285714 -0.62857143 -0.61428571 -0.6 -0.58571429 -0.57142857 -0.55714286 -0.54285714 -0.52857143 -0.51428571 -0.5 -0.48571429 -0.47142857 -0.45714286 -0.44285714 -0.42857143 -0.41428571 -0.4 -0.38571429 -0.37142857 -0.35714286 -0.34285714 -0.32857143 -0.31428571 -0.3 -0.28571429 -0.27142857 -0.25714286 -0.24285714 -0.22857143 -0.21428571 -0.2 -0.18571429 -0.17142857 -0.15714286 -0.14285714 -0.12857143 -0.11428571 -0.1 -0.08571429 -0.07142857 -0.05714286 -0.04285714 -0.02857143 -0.01428571 0 0 0 0 0 0
  line L9 (3.0131, 9.9639) -> (2.9153, 9.6417)
  arc A19 (2.1794, 9.2183) -> (2.9153, 9.6417) centre (2.322, 9.8216) ccw
  arc A20 (2.1794, 9.2183) -> (2.0361, 9.251) centre (0, 0) ccw
  arc A21 (1.5568, 9.9518) -> (2.0361, 9.251) centre (2.1694, 9.8565) ccw
  line L10 (1.5568, 9.9518) -> (1.6085, 10.2845)
  spline S10 degree 5 poles (1.6085, 10.2845) (1.6091, 10.2884) (1.6102, 10.2963) (1.6117, 10.3081) (1.6131, 10.3238) (1.6141, 10.3437) (1.6146, 10.3635) (1.6148, 10.3835) (1.6148, 10.4034) (1.6147, 10.4234) (1.6145, 10.4433) (1.6141, 10.4634) (1.6135, 10.4834) (1.6127, 10.5034) (1.6116, 10.5235) (1.6103, 10.5436) (1.6088, 10.5637) (1.6071, 10.5839) (1.6052, 10.604) (1.6033, 10.6242) (1.6012, 10.6444) (1.5989, 10.6646) (1.5965, 10.6848) (1.594, 10.705) (1.5913, 10.7252) (1.5884, 10.7455) (1.5854, 10.7657) (1.5823, 10.786) (1.5791, 10.8063) (1.5757, 10.8265) (1.5722, 10.8468) (1.5685, 10.8671) (1.5648, 10.8874) (1.5609, 10.9077) (1.5569, 10.928) (1.5527, 10.9483) (1.5485, 10.9687) (1.5441, 10.989) (1.5396, 11.0093) (1.535, 11.0297) (1.5303, 11.05) (1.5255, 11.0704) (1.5206, 11.0907) (1.5155, 11.1111) (1.5104, 11.1314) (1.5051, 11.1518) (1.4997, 11.1721) (1.4943, 11.1925) (1.4887, 11.2129) (1.483, 11.2332) (1.4772, 11.2536) (1.4713, 11.274) (1.4653, 11.2943) (1.4592, 11.3147) (1.453, 11.3351) (1.4467, 11.3554) (1.4403, 11.3758) (1.4338, 11.3961) (1.4272, 11.4165) (1.4205, 11.4369) (1.4137, 11.4572) (1.4068, 11.4776) (1.3998, 11.4979) (1.3928, 11.5183) (1.3856, 11.5386) (1.3783, 11.559) (1.3709, 11.5793) (1.3635, 11.5996) (1.3559, 11.62) (1.3483, 11.6403) (1.3405, 11.6606) (1.3343, 11.6769) (1.3295, 11.6891) (1.3264, 11.6972) (1.3248, 11.7012) knots 0 0 0 0 0 0 0.01428571 0.02857143 0.04285714 0.05714286 0.07142857 0.08571429 0.1 0.11428571 0.12857143 0.14285714 0.15714286 0.17142857 0.18571429 0.2 0.21428571 0.22857143 0.24285714 0.25714286 0.27142857 0.28571429 0.3 0.31428571 0.32857143 0.34285714 0.35714286 0.37142857 0.38571429 0.4 0.41428571 0.42857143 0.44285714 0.45714286 0.47142857 0.48571429 0.5 0.51428571 0.52857143 0.54285714 0.55714286 0.57142857 0.58571429 0.6 0.61428571 0.62857143 0.64285714 0.65714286 0.67142857 0.68571429 0.7 0.71428571 0.72857143 0.74285714 0.75714286 0.77142857 0.78571429 0.8 0.81428571 0.82857143 0.84285714 0.85714286 0.87142857 0.88571429 0.9 0.91428571 0.92857143 0.94285714 0.95714286 0.97142857 0.98571429 1 1 1 1 1 1
  arc A22 (1.3248, 11.7012) -> (0.434, 11.768) centre (0, 0) ccw
  spline S11 degree 5 poles (0.434, 11.768) (0.4318, 11.7642) (0.4275, 11.7567) (0.421, 11.7453) (0.4124, 11.7302) (0.4017, 11.7112) (0.3911, 11.6923) (0.3806, 11.6733) (0.3702, 11.6543) (0.3599, 11.6353) (0.3496, 11.6163) (0.3395, 11.5972) (0.3295, 11.5781) (0.3195, 11.5591) (0.3097, 11.54) (0.2999, 11.5208) (0.2903, 11.5017) (0.2807, 11.4826) (0.2713, 11.4634) (0.2619, 11.4442) (0.2526, 11.425) (0.2435, 11.4058) (0.2344, 11.3866) (0.2254, 11.3673) (0.2166, 11.3481) (0.2078, 11.3288) (0.1991, 11.3095) (0.1906, 11.2902) (0.1821, 11.2709) (0.1738, 11.2516) (0.1655, 11.2322) (0.1574, 11.2128) (0.1494, 11.1935) (0.1415, 11.1741) (0.1337, 11.1547) (0.126, 11.1353) (0.1184, 11.1158) (0.1109, 11.0964) (0.1036, 11.077) (0.0964, 11.0575) (0.0892, 11.038) (0.0823, 11.0185) (0.0754, 10.999) (0.0686, 10.9795) (0.062, 10.96) (0.0555, 10.9404) (0.0492, 10.9209) (0.0429, 10.9013) (0.0368, 10.8818) (0.0308, 10.8622) (0.025, 10.8426) (0.0193, 10.823) (0.0138, 10.8034) (0.0084, 10.7838) (0.0032, 10.7641) (-0.0019, 10.7445) (-0.0069, 10.7248) (-0.0117, 10.7052) (-0.0163, 10.6855) (-0.0208, 10.6659) (-0.0251, 10.6462) (-0.0292, 10.6265) (-0.033, 10.6068) (-0.0366, 10.5871) (-0.0399, 10.5673) (-0.0431, 10.5476) (-0.0462, 10.5279) (-0.0492, 10.5081) (-0.052, 10.4884) (-0.0544, 10.4687) (-0.0564, 10.4489) (-0.0573, 10.4331) (-0.0577, 10.4213) (-0.0577, 10.4133) (-0.0577, 10.4094) knots -1 -1 -1 -1 -1 -1 -0.98571429 -0.97142857 -0.95714286 -0.94285714 -0.92857143 -0.91428571 -0.9 -0.88571429 -0.87142857 -0.85714286 -0.84285714 -0.82857143 -0.81428571 -0.8 -0.78571429 -0.77142857 -0.75714286 -0.74285714 -0.72857143 -0.71428571 -0.7 -0.68571429 -0.67142857 -0.65714286 -0.64285714 -0.62857143 -0.61428571 -0.6 -0.58571429 -0.57142857 -0.55714286 -0.54285714 -0.52857143 -0.51428571 -0.5 -0.48571429 -0.47142857 -0.45714286 -0.44285714 -0.42857143 -0.41428571 -0.4 -0.38571429 -0.37142857 -0.35714286 -0.34285714 -0.32857143 -0.31428571 -0.3 -0.28571429 -0.27142857 -0.25714286 -0.24285714 -0.22857143 -0.21428571 -0.2 -0.18571429 -0.17142857 -0.15714286 -0.14285714 -0.12857143 -0.11428571 -0.1 -0.08571429 -0.07142857 -0.05714286 -0.04285714 -0.02857143 -0.01428571 0 0 0 0 0 0
  line L11 (-0.0577, 10.4094) -> (-0.0561, 10.0726)
  arc A23 (-0.6346, 9.4511) -> (-0.0561, 10.0726) centre (-0.6761, 10.0697) ccw
  arc A24 (-0.6346, 9.4511) -> (-0.7811, 9.4401) centre (0, 0) ccw
  arc A25 (-1.4457, 9.9685) -> (-0.7811, 9.4401) centre (-0.8322, 10.058) ccw
  line L12 (-1.4457, 9.9685) -> (-1.4944, 10.3017)
  spline S12 degree 5 poles (-1.4944, 10.3017) (-1.4949, 10.3056) (-1.4962, 10.3135) (-1.4983, 10.3251) (-1.5016, 10.3406) (-1.5065, 10.3599) (-1.5118, 10.379) (-1.5175, 10.3981) (-1.5234, 10.4172) (-1.5294, 10.4362) (-1.5355, 10.4553) (-1.5417, 10.4743) (-1.5482, 10.4932) (-1.5549, 10.5121) (-1.5619, 10.531) (-1.5691, 10.5498) (-1.5764, 10.5686) (-1.584, 10.5874) (-1.5917, 10.6061) (-1.5995, 10.6248) (-1.6074, 10.6434) (-1.6155, 10.6621) (-1.6238, 10.6807) (-1.6322, 10.6992) (-1.6407, 10.7178) (-1.6494, 10.7363) (-1.6582, 10.7547) (-1.6672, 10.7732) (-1.6763, 10.7916) (-1.6855, 10.81) (-1.6948, 10.8283) (-1.7043, 10.8466) (-1.7139, 10.8649) (-1.7236, 10.8832) (-1.7334, 10.9014) (-1.7433, 10.9196) (-1.7534, 10.9378) (-1.7635, 10.9559) (-1.7738, 10.974) (-1.7842, 10.9921) (-1.7947, 11.0102) (-1.8053, 11.0282) (-1.816, 11.0462) (-1.8268, 11.0641) (-1.8378, 11.0821) (-1.8488, 11.1) (-1.8599, 11.1179) (-1.8712, 11.1357) (-1.8825, 11.1535) (-1.8939, 11.1713) (-1.9055, 11.189) (-1.9171, 11.2068) (-1.9288, 11.2245) (-1.9407, 11.2421) (-1.9526, 11.2598) (-1.9646, 11.2774) (-1.9768, 11.2949) (-1.989, 11.3125) (-2.0013, 11.33) (-2.0137, 11.3475) (-2.0262, 11.3649) (-2.0388, 11.3823) (-2.0514, 11.3997) (-2.0642, 11.4171) (-2.0771, 11.4344) (-2.09, 11.4517) (-2.103, 11.469) (-2.1162, 11.4862) (-2.1294, 11.5034) (-2.1427, 11.5206) (-2.156, 11.5377) (-2.1668, 11.5514) (-2.1749, 11.5616) (-2.1804, 11.5685) (-2.1831, 11.5719) knots 0 0 0 0 0 0 0.01428571 0.02857143 0.04285714 0.05714286 0.07142857 0.08571429 0.1 0.11428571 0.12857143 0.14285714 0.15714286 0.17142857 0.18571429 0.2 0.21428571 0.22857143 0.24285714 0.25714286 0.27142857 0.28571429 0.3 0.31428571 0.32857143 0.34285714 0.35714286 0.37142857 0.38571429 0.4 0.41428571 0.42857143 0.44285714 0.45714286 0.47142857 0.48571429 0.5 0.51428571 0.52857143 0.54285714 0.55714286 0.57142857 0.58571429 0.6 0.61428571 0.62857143 0.64285714 0.65714286 0.67142857 0.68571429 0.7 0.71428571 0.72857143 0.74285714 0.75714286 0.77142857 0.78571429 0.8 0.81428571 0.82857143 0.84285714 0.85714286 0.87142857 0.88571429 0.9 0.91428571 0.92857143 0.94285714 0.95714286 0.97142857 0.98571429 1 1 1 1 1 1
  arc A26 (-2.1831, 11.5719) -> (-3.0539, 11.3731) centre (0, 0) ccw
  spline S13 degree 5 poles (-3.0539, 11.3731) (-3.0549, 11.3689) (-3.0568, 11.3603) (-3.0597, 11.3476) (-3.0635, 11.3306) (-3.0681, 11.3093) (-3.0726, 11.2881) (-3.0771, 11.2669) (-3.0814, 11.2456) (-3.0857, 11.2244) (-3.0898, 11.2032) (-3.0939, 11.182) (-3.0979, 11.1609) (-3.1018, 11.1397) (-3.1055, 11.1185) (-3.1092, 11.0974) (-3.1128, 11.0763) (-3.1163, 11.0552) (-3.1197, 11.0341) (-3.123, 11.013) (-3.1262, 10.9919) (-3.1293, 10.9708) (-3.1323, 10.9498) (-3.1352, 10.9288) (-3.138, 10.9077) (-3.1407, 10.8867) (-3.1432, 10.8658) (-3.1457, 10.8448) (-3.1481, 10.8238) (-3.1504, 10.8029) (-3.1526, 10.782) (-3.1546, 10.7611) (-3.1566, 10.7402) (-3.1584, 10.7194) (-3.1602, 10.6985) (-3.1618, 10.6777) (-3.1633, 10.6569) (-3.1647, 10.6361) (-3.166, 10.6154) (-3.1672, 10.5946) (-3.1682, 10.5739) (-3.1692, 10.5532) (-3.17, 10.5326) (-3.1707, 10.512) (-3.1712, 10.4913) (-3.1717, 10.4708) (-3.172, 10.4502) (-3.1722, 10.4297) (-3.1723, 10.4092) (-3.1722, 10.3887) (-3.172, 10.3683) (-3.1717, 10.3479) (-3.1712, 10.3275) (-3.1705, 10.3072) (-3.1698, 10.2869) (-3.1688, 10.2666) (-3.1678, 10.2464) (-3.1666, 10.2261) (-3.1652, 10.206) (-3.1637, 10.1859) (-3.162, 10.1658) (-3.1601, 10.1458) (-3.1579, 10.1258) (-3.1555, 10.1059) (-3.1529, 10.0861) (-3.1502, 10.0663) (-3.1473, 10.0465) (-3.1443, 10.0268) (-3.1412, 10.0071) (-3.1377, 9.9876) (-3.1337, 9.9681) (-3.13, 9.9527) (-3.1268, 9.9413) (-3.1246, 9.9337) (-3.1234, 9.9299) knots -1 -1 -1 -1 -1 -1 -0.98571429 -0.97142857 -0.95714286 -0.94285714 -0.92857143 -0.91428571 -0.9 -0.88571429 -0.87142857 -0.85714286 -0.84285714 -0.82857143 -0.81428571 -0.8 -0.78571429 -0.77142857 -0.75714286 -0.74285714 -0.72857143 -0.71428571 -0.7 -0.68571429 -0.67142857 -0.65714286 -0.64285714 -0.62857143 -0.61428571 -0.6 -0.58571429 -0.57142857 -0.55714286 -0.54285714 -0.52857143 -0.51428571 -0.5 -0.48571429 -0.47142857 -0.45714286 -0.44285714 -0.42857143 -0.41428571 -0.4 -0.38571429 -0.37142857 -0.35714286 -0.34285714 -0.32857143 -0.31428571 -0.3 -0.28571429 -0.27142857 -0.25714286 -0.24285714 -0.22857143 -0.21428571 -0.2 -0.18571429 -0.17142857 -0.15714286 -0.14285714 -0.12857143 -0.11428571 -0.1 -0.08571429 -0.07142857 -0.05714286 -0.04285714 -0.02857143 -0.01428571 0 0 0 0 0 0
  line L13 (-3.1234, 9.9299) -> (-3.0226, 9.6086)
  arc A27 (-3.3922, 8.8442) -> (-3.0226, 9.6086) centre (-3.6142, 9.4231) ccw
  arc A28 (-3.3922, 8.8442) -> (-3.5289, 8.7905) centre (0, 0) ccw
  arc A29 (-4.3198, 9.0995) -> (-3.5289, 8.7905) centre (-3.7599, 9.3659) ccw
  line L14 (-4.3198, 9.0995) -> (-4.4645, 9.4036)
  spline S14 degree 5 poles (-4.4645, 9.4036) (-4.4662, 9.4071) (-4.4696, 9.4143) (-4.4751, 9.4248) (-4.4829, 9.4386) (-4.4932, 9.4556) (-4.5039, 9.4723) (-4.515, 9.4889) (-4.5262, 9.5053) (-4.5376, 9.5218) (-4.549, 9.5382) (-4.5606, 9.5545) (-4.5724, 9.5707) (-4.5844, 9.5868) (-4.5966, 9.6028) (-4.609, 9.6186) (-4.6215, 9.6344) (-4.6343, 9.6501) (-4.6472, 9.6657) (-4.6601, 9.6813) (-4.6732, 9.6968) (-4.6865, 9.7122) (-4.6998, 9.7275) (-4.7133, 9.7428) (-4.727, 9.758) (-4.7407, 9.7731) (-4.7546, 9.7882) (-4.7686, 9.8031) (-4.7827, 9.8181) (-4.7969, 9.8329) (-4.8112, 9.8477) (-4.8257, 9.8624) (-4.8402, 9.8771) (-4.8549, 9.8917) (-4.8696, 9.9062) (-4.8845, 9.9206) (-4.8994, 9.935) (-4.9145, 9.9494) (-4.9297, 9.9637) (-4.9449, 9.9779) (-4.9603, 9.992) (-4.9757, 10.0061) (-4.9913, 10.0202) (-5.0069, 10.0341) (-5.0226, 10.048) (-5.0384, 10.0619) (-5.0543, 10.0757) (-5.0703, 10.0894) (-5.0864, 10.1031) (-5.1026, 10.1167) (-5.1189, 10.1303) (-5.1352, 10.1438) (-5.1516, 10.1572) (-5.1681, 10.1706) (-5.1847, 10.184) (-5.2014, 10.1972) (-5.2182, 10.2105) (-5.235, 10.2236) (-5.2519, 10.2367) (-5.2689, 10.2498) (-5.286, 10.2628) (-5.3032, 10.2757) (-5.3204, 10.2886) (-5.3377, 10.3014) (-5.3551, 10.3142) (-5.3726, 10.3269) (-5.3901, 10.3395) (-5.4078, 10.3521) (-5.4254, 10.3647) (-5.4432, 10.3772) (-5.4611, 10.3896) (-5.4754, 10.3995) (-5.4862, 10.4069) (-5.4934, 10.4118) (-5.497, 10.4143) knots 0 0 0 0 0 0 0.01428571 0.02857143 0.04285714 0.05714286 0.07142857 0.08571429 0.1 0.11428571 0.12857143 0.14285714 0.15714286 0.17142857 0.18571429 0.2 0.21428571 0.22857143 0.24285714 0.25714286 0.27142857 0.28571429 0.3 0.31428571 0.32857143 0.34285714 0.35714286 0.37142857 0.38571429 0.4 0.41428571 0.42857143 0.44285714 0.45714286 0.47142857 0.48571429 0.5 0.51428571 0.52857143 0.54285714 0.55714286 0.57142857 0.58571429 0.6 0.61428571 0.62857143 0.64285714 0.65714286 0.67142857 0.68571429 0.7 0.71428571 0.72857143 0.74285714 0.75714286 0.77142857 0.78571429 0.8 0.81428571 0.82857143 0.84285714 0.85714286 0.87142857 0.88571429 0.9 0.91428571 0.92857143 0.94285714 0.95714286 0.97142857 0.98571429 1 1 1 1 1 1
  arc A30 (-5.497, 10.4143) -> (-6.2706, 9.9677) centre (0, 0) ccw
  spline S15 degree 5 poles (-6.2706, 9.9677) (-6.2702, 9.9633) (-6.2696, 9.9546) (-6.2685, 9.9416) (-6.2671, 9.9242) (-6.2653, 9.9025) (-6.2634, 9.8809) (-6.2613, 9.8593) (-6.2592, 9.8378) (-6.2571, 9.8162) (-6.2548, 9.7948) (-6.2524, 9.7733) (-6.25, 9.7519) (-6.2474, 9.7305) (-6.2448, 9.7092) (-6.2421, 9.6879) (-6.2393, 9.6667) (-6.2364, 9.6455) (-6.2334, 9.6243) (-6.2304, 9.6032) (-6.2272, 9.5821) (-6.224, 9.5611) (-6.2206, 9.5401) (-6.2172, 9.5191) (-6.2137, 9.4982) (-6.2101, 9.4773) (-6.2063, 9.4565) (-6.2025, 9.4358) (-6.1986, 9.415) (-6.1946, 9.3944) (-6.1906, 9.3737) (-6.1864, 9.3532) (-6.1821, 9.3326) (-6.1777, 9.3122) (-6.1732, 9.2917) (-6.1686, 9.2714) (-6.1639, 9.251) (-6.1592, 9.2308) (-6.1543, 9.2106) (-6.1493, 9.1904) (-6.1442, 9.1703) (-6.139, 9.1503) (-6.1337, 9.1303) (-6.1283, 9.1104) (-6.1227, 9.0905) (-6.1171, 9.0707) (-6.1113, 9.051) (-6.1055, 9.0313) (-6.0995, 9.0117) (-6.0934, 8.9921) (-6.0872, 8.9727) (-6.0809, 8.9533) (-6.0744, 8.9339) (-6.0678, 8.9147) (-6.061, 8.8955) (-6.0542, 8.8764) (-6.0472, 8.8574) (-6.0401, 8.8385) (-6.0329, 8.8196) (-6.0255, 8.8008) (-6.018, 8.7821) (-6.0102, 8.7636) (-6.0023, 8.7451) (-5.9941, 8.7268) (-5.9858, 8.7086) (-5.9773, 8.6905) (-5.9688, 8.6725) (-5.9601, 8.6545) (-5.9513, 8.6367) (-5.9422, 8.619) (-5.9327, 8.6016) (-5.9246, 8.588) (-5.9182, 8.5779) (-5.9137, 8.5714) (-5.9115, 8.5681) knots -1 -1 -1 -1 -1 -1 -0.98571429 -0.97142857 -0.95714286 -0.94285714 -0.92857143 -0.91428571 -0.9 -0.88571429 -0.87142857 -0.85714286 -0.84285714 -0.82857143 -0.81428571 -0.8 -0.78571429 -0.77142857 -0.75714286 -0.74285714 -0.72857143 -0.71428571 -0.7 -0.68571429 -0.67142857 -0.65714286 -0.64285714 -0.62857143 -0.61428571 -0.6 -0.58571429 -0.57142857 -0.55714286 -0.54285714 -0.52857143 -0.51428571 -0.5 -0.48571429 -0.47142857 -0.45714286 -0.44285714 -0.42857143 -0.41428571 -0.4 -0.38571429 -0.37142857 -0.35714286 -0.34285714 -0.32857143 -0.31428571 -0.3 -0.28571429 -0.27142857 -0.25714286 -0.24285714 -0.22857143 -0.21428571 -0.2 -0.18571429 -0.17142857 -0.15714286 -0.14285714 -0.12857143 -0.11428571 -0.1 -0.08571429 -0.07142857 -0.05714286 -0.04285714 -0.02857143 -0.01428571 0 0 0 0 0 0
  line L15 (-5.9115, 8.5681) -> (-5.7205, 8.2908)
  arc A31 (-5.8483, 7.4514) -> (-5.7205, 8.2908) centre (-6.2311, 7.9391) ccw
  arc A32 (-5.8483, 7.4514) -> (-5.9632, 7.3598) centre (0, 0) ccw
  arc A33 (-6.81, 7.422) -> (-5.9632, 7.3598) centre (-6.3535, 7.8415) ccw
  line L16 (-6.81, 7.422) -> (-7.0379, 7.6699)
  spline S16 degree 5 poles (-7.0379, 7.6699) (-7.0405, 7.6728) (-7.046, 7.6786) (-7.0543, 7.687) (-7.0658, 7.698) (-7.0806, 7.7111) (-7.0958, 7.7239) (-7.1113, 7.7365) (-7.1269, 7.7489) (-7.1426, 7.7613) (-7.1583, 7.7736) (-7.1742, 7.7857) (-7.1902, 7.7978) (-7.2064, 7.8096) (-7.2228, 7.8213) (-7.2393, 7.8328) (-7.256, 7.8442) (-7.2728, 7.8554) (-7.2897, 7.8665) (-7.3067, 7.8776) (-7.3238, 7.8885) (-7.341, 7.8993) (-7.3583, 7.9101) (-7.3757, 7.9207) (-7.3932, 7.9312) (-7.4108, 7.9416) (-7.4285, 7.9519) (-7.4463, 7.9621) (-7.4641, 7.9721) (-7.4821, 7.9821) (-7.5002, 7.992) (-7.5183, 8.0019) (-7.5365, 8.0116) (-7.5548, 8.0212) (-7.5732, 8.0307) (-7.5916, 8.0402) (-7.6102, 8.0495) (-7.6288, 8.0588) (-7.6475, 8.068) (-7.6663, 8.077) (-7.6851, 8.086) (-7.704, 8.095) (-7.723, 8.1038) (-7.7421, 8.1125) (-7.7612, 8.1212) (-7.7804, 8.1298) (-7.7997, 8.1383) (-7.819, 8.1467) (-7.8384, 8.155) (-7.8579, 8.1633) (-7.8774, 8.1714) (-7.897, 8.1795) (-7.9167, 8.1875) (-7.9364, 8.1955) (-7.9562, 8.2033) (-7.976, 8.2111) (-7.9959, 8.2188) (-8.0159, 8.2264) (-8.0359, 8.2339) (-8.056, 8.2414) (-8.0762, 8.2487) (-8.0964, 8.256) (-8.1167, 8.2633) (-8.137, 8.2704) (-8.1574, 8.2775) (-8.1778, 8.2845) (-8.1983, 8.2914) (-8.2188, 8.2983) (-8.2395, 8.305) (-8.2601, 8.3117) (-8.2808, 8.3183) (-8.2974, 8.3236) (-8.3099, 8.3275) (-8.3183, 8.3301) (-8.3224, 8.3313) knots 0 0 0 0 0 0 0.01428571 0.02857143 0.04285714 0.05714286 0.07142857 0.08571429 0.1 0.11428571 0.12857143 0.14285714 0.15714286 0.17142857 0.18571429 0.2 0.21428571 0.22857143 0.24285714 0.25714286 0.27142857 0.28571429 0.3 0.31428571 0.32857143 0.34285714 0.35714286 0.37142857 0.38571429 0.4 0.41428571 0.42857143 0.44285714 0.45714286 0.47142857 0.48571429 0.5 0.51428571 0.52857143 0.54285714 0.55714286 0.57142857 0.58571429 0.6 0.61428571 0.62857143 0.64285714 0.65714286 0.67142857 0.68571429 0.7 0.71428571 0.72857143 0.74285714 0.75714286 0.77142857 0.78571429 0.8 0.81428571 0.82857143 0.84285714 0.85714286 0.87142857 0.88571429 0.9 0.91428571 0.92857143 0.94285714 0.95714286 0.97142857 0.98571429 1 1 1 1 1 1
  arc A34 (-8.3224, 8.3313) -> (-8.93, 7.6766) centre (0, 0) ccw
  spline S17 degree 5 poles (-8.93, 7.6766) (-8.9284, 7.6725) (-8.9252, 7.6644) (-8.9204, 7.6522) (-8.9139, 7.636) (-8.9058, 7.6159) (-8.8975, 7.5958) (-8.8893, 7.5757) (-8.8809, 7.5558) (-8.8725, 7.5358) (-8.864, 7.516) (-8.8554, 7.4962) (-8.8467, 7.4764) (-8.838, 7.4568) (-8.8292, 7.4372) (-8.8203, 7.4176) (-8.8114, 7.3981) (-8.8024, 7.3787) (-8.7933, 7.3594) (-8.7842, 7.3401) (-8.7749, 7.3209) (-8.7656, 7.3017) (-8.7562, 7.2827) (-8.7468, 7.2637) (-8.7373, 7.2447) (-8.7277, 7.2258) (-8.718, 7.207) (-8.7082, 7.1883) (-8.6984, 7.1697) (-8.6885, 7.1511) (-8.6785, 7.1326) (-8.6684, 7.1142) (-8.6583, 7.0958) (-8.648, 7.0775) (-8.6377, 7.0593) (-8.6274, 7.0412) (-8.6169, 7.0232) (-8.6063, 7.0052) (-8.5957, 6.9874) (-8.585, 6.9696) (-8.5742, 6.9519) (-8.5633, 6.9342) (-8.5524, 6.9167) (-8.5413, 6.8993) (-8.5302, 6.8819) (-8.519, 6.8647) (-8.5076, 6.8475) (-8.4962, 6.8304) (-8.4848, 6.8135) (-8.4732, 6.7966) (-8.4615, 6.7798) (-8.4497, 6.7631) (-8.4378, 6.7466) (-8.4259, 6.7301) (-8.4138, 6.7138) (-8.4016, 6.6976) (-8.3893, 6.6815) (-8.3769, 6.6654) (-8.3645, 6.6495) (-8.3519, 6.6338) (-8.3392, 6.6181) (-8.3263, 6.6027) (-8.3133, 6.5874) (-8.3001, 6.5723) (-8.2868, 6.5574) (-8.2733, 6.5426) (-8.2598, 6.5279) (-8.2463, 6.5133) (-8.2326, 6.4988) (-8.2187, 6.4846) (-8.2045, 6.4708) (-8.1927, 6.4601) (-8.1836, 6.4524) (-8.1775, 6.4475) (-8.1744, 6.445) knots -1 -1 -1 -1 -1 -1 -0.98571429 -0.97142857 -0.95714286 -0.94285714 -0.92857143 -0.91428571 -0.9 -0.88571429 -0.87142857 -0.85714286 -0.84285714 -0.82857143 -0.81428571 -0.8 -0.78571429 -0.77142857 -0.75714286 -0.74285714 -0.72857143 -0.71428571 -0.7 -0.68571429 -0.67142857 -0.65714286 -0.64285714 -0.62857143 -0.61428571 -0.6 -0.58571429 -0.57142857 -0.55714286 -0.54285714 -0.52857143 -0.51428571 -0.5 -0.48571429 -0.47142857 -0.45714286 -0.44285714 -0.42857143 -0.41428571 -0.4 -0.38571429 -0.37142857 -0.35714286 -0.34285714 -0.32857143 -0.31428571 -0.3 -0.28571429 -0.27142857 -0.25714286 -0.24285714 -0.22857143 -0.21428571 -0.2 -0.18571429 -0.17142857 -0.15714286 -0.14285714 -0.12857143 -0.11428571 -0.1 -0.08571429 -0.07142857 -0.05714286 -0.04285714 -0.02857143 -0.01428571 0 0 0 0 0 0
  line L17 (-8.1744, 6.445) -> (-7.9101, 6.2363)
  arc A35 (-7.7848, 5.3965) -> (-7.9101, 6.2363) centre (-8.2944, 5.7498) ccw
  arc A36 (-7.7848, 5.3965) -> (-7.8676, 5.2751) centre (0, 0) ccw
  arc A37 (-8.6951, 5.0849) -> (-7.8676, 5.2751) centre (-8.3826, 5.6204) ccw
  line L18 (-8.6951, 5.0849) -> (-8.9859, 5.2547)